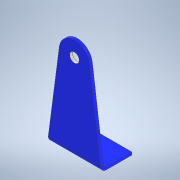
# Autodesk Inventor part: soporte_barra
Saved by Autodesk Inventor 2021 (Build 250183000, 183)
## iProperties
Created: 2021-04-16
Part Number: soporte_barra
Material: Genérico
Document SubType Name: Chapa
Designer: Leonardo Fabio Mercado Benítez
Density: 1 g/cm^3
Sheet Metal Rule: Por defecto_mm
Appearance: Valor por defecto
Author: Leonardo Fabio Mercado Benítez
Autodesk Inventor part; units mm, degrees
ref_plane "YZ Plane" through (0, 0, 0) normal (1, 0, 0) x (0, 1, 0)
ref_plane "XZ Plane" through (0, 0, 0) normal (0, 1, 0) x (-1, 0, 0)
ref_plane "XY Plane" through (0, 0, 0) normal (0, 0, 1) x (1, 0, 0)
sketch "Boceto1" plane through (0, 0, 0) normal (0, 1, 0) x (-1, 0, 0)
  line L0 (-17.5, 8.5) -> (17.5, 8.5)
  line L1 (17.5, 8.5) -> (17.5, -8.5)
  line L2 (17.5, -8.5) -> (-17.5, -8.5)
  line L3 (-17.5, -8.5) -> (-17.5, 8.5)
  line L4 (-17.5, 8.5) -> (17.5, -8.5) construction
  line L5 (17.5, 8.5) -> (-17.5, -8.5) construction
  point P0 (0, 0)
  dimension "d0" = 35
  dimension "d1" = 17
  measures "d0" distance of L1.end L2.end
  measures "d1" distance of L0.end L1.end
extrude "Placa1" add sketch "Boceto1" along normal blind 1.9
sketch "Boceto2" plane through (17.5, 3.8, 10.4) normal (0, 0, 1) x (1, 0, 0)
  line L0 (-35, 0) -> (0, 0)
  line L1 (0, 0) -> (0, 66.2)
  line L2 (0, 66.2) -> (-35, 66.2)
  line L3 (-35, 66.2) -> (-35, 0)
  constraints: 6 end point, 1 horizontal, 1 perpendicular, 1 vertical
edge flange "Pestaña1" height 70 angle 90 thickness 1.9 bend radius 1.9 thickness toward (0, 0, 1) relief straight relief width 1.9 relief depth 0.95 edges at (0, 1.9, 8.5) wall of the first edge with corners at (-17.5, 3.8, 10.4) (17.5, 3.8, 10.4) (17.5, 70, 10.4) (-17.5, 70, 10.4)
bend "Doblez1"
corner "Esquina1"
sketch "Boceto5" plane through (-17.5, 70, 12.3) normal (0, 0, 1) x (1, 0, 0)
  arc A0 (27.5986, -10.5274) -> (7.4014, -10.5274) centre (17.5, -11.87) ccw
  line L0 (0, -66.2) -> (7.4014, -10.5274)
  line L1 (35, -66.2) -> (27.5986, -10.5274)
  line L2 (0, 0) -> (35, 0) projected
  line L3 (0, -66.2) -> (0, 0)
  line L4 (0, 0) -> (35, 0)
  line L5 (35, 0) -> (35, -66.2)
  point P0 (17.5, -70)
  dimension "d21" = 20.375
  constraints: 10 end point, 3 perpendicular, 2 point on circle, 2 tangent, 1 centre point
  measures "d21" diameter of A0
extrude "Cortar2" cut sketch "Boceto5" against normal blind 1.9
sketch "Boceto6" plane through (-17.5, 3.8, 12.3) normal (0, 0, 1) x (1, 0, 0)
  line L0 (7.4014, 55.6726) -> (0, 0) projected
  line L1 (0, 0) -> (35, 0) projected
  line L2 (35, 0) -> (27.5986, 55.6726) projected
  arc A0 (27.5986, 55.6726) -> (7.4014, 55.6726) centre (17.5, 54.33) ccw projected
  circle A1 centre (17.5, 54.33) radius 3.175
  point P0 (17.5, -3.8)
  dimension "d26" = 6.35
  constraints: 1 centre point, 1 coincident
  measures "d26" diameter of A1
extrude "Cortar3" cut sketch "Boceto6" against normal blind 1.9 contours A1
equation "\"d24\" = Grosor"
equation "\"d27\" = Grosor"
equation "\"d2\" = Grosor"
equation "\"d3\" = Anchura_desahogo_plegado"
equation "\"d4\" = Profundidad_desahogo_plegado"
equation "\"d5\" = Remanente_mínimo"
equation "\"d6\" = Radiodetransición"
equation "\"d9\" = Radio_pliegue"
equation "\"d10\" = Tamaño_destalonado"
equation "\"d11\" = TamañoSeparación"
equation "\"d12\" = Tamaño_de_radio_de_Jacobi"
equation "\"Radio_pliegue\" = Grosor"
equation "\"Anchura_desahogo_plegado\" = Grosor"
equation "\"Profundidad_desahogo_plegado\" = 0.5 * Grosor"
equation "\"Tamaño_destalonado\" = 4 * Grosor"
equation "\"Remanente_mínimo\" = 2 * Grosor"
equation "\"Radiodetransición\" = Radio_pliegue"
equation "\"Tamaño_de_radio_de_Jacobi\" = Radio_pliegue"
equation "\"TamañoSeparación\" = Grosor"
equation "\"Grosor\" = 1.9"
